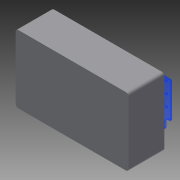
# Autodesk Inventor part: boks
Saved by Autodesk Inventor 2015 (Build 190159000, 159)
## iProperties
Created: 2015-07-23
Part Number: boks
Material: Generic
Document SubType Name: Modeling
Designer: Simen
Density: 1 g/cm^3
Appearance: Default
Author: Simen
Autodesk Inventor part; units mm, degrees
ref_plane "YZ Plane" through (0, 0, 0) normal (1, 0, 0) x (0, 1, 0)
ref_plane "XZ Plane" through (0, 0, 0) normal (0, 1, 0) x (-1, 0, 0)
ref_plane "XY Plane" through (0, 0, 0) normal (0, 0, 1) x (1, 0, 0)
sketch "Sketch1" plane through (0, 0, 0) normal (0, 1, 0) x (-1, 0, 0)
  line L0 (0, 0) -> (200, 0)
  line L1 (200, 0) -> (200, -120)
  line L2 (200, -120) -> (0, -120)
  line L3 (0, -120) -> (0, 0)
  dimension "d0" = 200
  dimension "d1" = 120
  constraints: 8 end point, 2 parallel, 1 horizontal, 1 perpendicular
  measures "d0" distance of L1.end L2.end
  measures "d1" distance of L0.end L1.end
extrude "Extrusion1" add sketch "Sketch1" along normal blind 3
sketch "Sketch2" plane through (0, 3, 0) normal (0, 1, 0) x (1, 0, 0)
  line L0 (-200, 0) -> (0, 0) projected
  line L1 (0, 0) -> (0, 120) projected
  line L2 (0, 120) -> (-200, 120) projected
  line L3 (-200, 120) -> (-200, 0) projected
  line L4 (-181.5, 116.5) -> (-18.5, 116.5)
  line L5 (-3.5, 92.5) -> (-3.5, 27.5)
  line L6 (-18.5, 3.5) -> (-181.5, 3.5)
  line L7 (-196.5, 27.5) -> (-196.5, 92.5)
  line L8 (-196.5, 3.5) -> (-186.5, 3.5)
  line L9 (-186.5, 8.5) -> (-186.5, 17.5)
  line L10 (-191.5, 22.5) -> (-191.5, 22.5)
  line L11 (-196.5, 22.5) -> (-196.5, 3.5)
  line L12 (-196.5, 116.5) -> (-186.5, 116.5)
  line L13 (-186.5, 111.5) -> (-186.5, 102.5)
  line L14 (-191.5, 97.5) -> (-191.5, 97.5)
  line L15 (-196.5, 97.5) -> (-196.5, 116.5)
  line L16 (-3.5, 116.5) -> (-13.5, 116.5)
  line L17 (-13.5, 111.5) -> (-13.5, 102.5)
  line L18 (-8.5, 97.5) -> (-8.5, 97.5)
  line L19 (-3.5, 97.5) -> (-3.5, 116.5)
  line L20 (-3.5, 3.5) -> (-13.5, 3.5)
  line L21 (-13.5, 8.5) -> (-13.5, 17.5)
  line L22 (-8.5, 22.5) -> (-8.5, 22.5)
  line L23 (-3.5, 22.5) -> (-3.5, 3.5)
  arc A0 (-3.5, 92.5) -> (-8.5, 97.5) centre (-8.5, 92.5) ccw
  arc A1 (-13.5, 111.5) -> (-18.5, 116.5) centre (-18.5, 111.5) ccw
  arc A2 (-8.5, 22.5) -> (-3.5, 27.5) centre (-8.5, 27.5) ccw
  arc A3 (-18.5, 3.5) -> (-13.5, 8.5) centre (-18.5, 8.5) ccw
  arc A4 (-186.5, 8.5) -> (-181.5, 3.5) centre (-181.5, 8.5) ccw
  arc A5 (-196.5, 27.5) -> (-191.5, 22.5) centre (-191.5, 27.5) ccw
  arc A6 (-191.5, 97.5) -> (-196.5, 92.5) centre (-191.5, 92.5) ccw
  arc A7 (-181.5, 116.5) -> (-186.5, 111.5) centre (-181.5, 111.5) ccw
  arc A8 (-191.5, 97.5) -> (-186.5, 102.5) centre (-191.5, 102.5) ccw
  arc A9 (-186.5, 17.5) -> (-191.5, 22.5) centre (-191.5, 17.5) ccw
  arc A10 (-8.5, 22.5) -> (-13.5, 17.5) centre (-8.5, 17.5) ccw
  arc A11 (-13.5, 102.5) -> (-8.5, 97.5) centre (-8.5, 102.5) ccw
  line L24 (-196.5, 116.5) -> (-200, 116.5)
  line L25 (-196.5, 3.5) -> (-200, 3.5)
  line L26 (-3.5, 3.5) -> (-3.5, 0)
  line L27 (-3.5, 116.5) -> (-3.5, 120)
  line L28 (-196.5, 3.5) -> (-196.5, 0)
  point P0 (-186.5, 22.5)
  point P1 (-186.5, 97.5)
  point P2 (-13.5, 97.5)
  point P3 (-13.5, 22.5)
  dimension "d4" = 3.5
  dimension "d7" = 10
  dimension "d8" = 19
  dimension "d9" = 10
  dimension "d10" = 19
  dimension "d11" = 10
  dimension "d12" = 19
  dimension "d13" = 10
  dimension "d14" = 19
  dimension "d15" = 5
  dimension "d16" = 5
  dimension "d17" = 5
  dimension "d18" = 5
  dimension "d19" = 5
  dimension "d20" = 5
  dimension "d21" = 5
  dimension "d22" = 5
  dimension "d23" = 5
  dimension "d73" = 3.5
  dimension "d74" = 3.5
  dimension "d75" = 3.5
  dimension "d78" = 3.5
  constraints: 50 end point, 29 point on line, 24 point on circle, 24 tangent, 12 centre point, 8 parallel, 8 perpendicular, 4 horizontal, 3 equal radius, 1 vertical, 1 other
  measures "d4" distance between parallel lines of L2 L4
  measures "d7" distance of L11.start point (-186.5, 22.5)
  measures "d8" distance of L8.end point (-186.5, 22.5)
  measures "d9" distance of point (-186.5, 97.5) L15.start
  measures "d10" distance of L12.end point (-186.5, 97.5)
  measures "d11" distance of L19.start point (-13.5, 97.5)
  measures "d12" distance of point (-13.5, 97.5) L16.end
  measures "d13" distance of point (-13.5, 22.5) L23.start
  measures "d14" distance of L20.end point (-13.5, 22.5)
  measures "d15" radius of A0
  measures "d16" radius of A1
  measures "d17" radius of A2
  measures "d18" radius of A3
  measures "d19" radius of A4
  measures "d20" radius of A5
  measures "d21" radius of A6
  measures "d22" radius of A7
  measures "d23" radius of A8
  measures "d73" distance of L12.start L24.end
  measures "d74" distance of L8.start L25.end
  measures "d75" distance of L20.start L26.end
  measures "d78" distance of L8.start L28.end
extrude "Extrusion2" add sketch "Sketch2" along normal blind 60
sketch "Sketch3" plane through (0, 3, 0) normal (0, 1, 0) x (1, 0, 0)
  line L0 (-200, 120) -> (-200, 105)
  line L1 (-200, 120) -> (-200, 0) projected
  line L2 (0, 120) -> (0, 0) projected
  line L3 (0, 0) -> (0, 15)
  line L4 (-181.5, 3.5) -> (-18.5, 3.5) projected
  circle A0 centre (-180, 105) radius 1.5
  line L5 (-180, 105) -> (-158, 105)
  circle A1 centre (-158, 105) radius 1.5
  circle A2 centre (-187.5, 60) radius 1.5
  line L6 (-187.5, 60) -> (-187.5, 80)
  line L7 (-187.5, 60) -> (-187.5, 40)
  circle A3 centre (-187.5, 40) radius 1.5
  circle A4 centre (-187.5, 80) radius 1.5
  line L8 (-200, 0) -> (-200, 120) projected
  line L9 (-187.5, 60) -> (-12.5, 60)
  circle A5 centre (-12.5, 60) radius 1.5
  line L10 (0, 120) -> (-200, 120) projected
  line L11 (-100, 120) -> (-100, 0)
  line L12 (0, 0) -> (-200, 0) projected
  circle A6 centre (-20, 105) radius 1.5
  line L13 (-180, 105) -> (-181.5, 105)
  line L14 (-184, 106) -> (-200, 106)
  line L15 (-180, 105) -> (-159.5, 105)
  line L16 (-180, 15) -> (-20, 15)
  circle A7 centre (-180, 15) radius 1.5
  line L17 (-84.857, 105) -> (-84.857, 15)
  line L18 (-158, 105) -> (-20, 105)
  circle A8 centre (-20, 15) radius 1.5
  line L19 (-12.5, 60) -> (-12.5, 40)
  line L20 (-12.5, 60) -> (-12.5, 80)
  circle A9 centre (-12.5, 80) radius 1.5
  circle A10 centre (-12.5, 40) radius 1.5
  line L21 (-180, 105) -> (-20, 105)
  line L22 (-13.5, 111.5) -> (-13.5, 102.5) projected
  point P0 (-100, 60)
  point P1 (-100, 15)
  point P2 (-84.857, 60)
  point P3 (-100, 105)
  dimension "d35" = 3
  dimension "d37" = 3
  dimension "d24" = 15
  dimension "d36" = 22
  dimension "d41" = 3
  dimension "d44" = 20
  dimension "d45" = 20
  dimension "d54" = 175
  dimension "d55" = 3
  dimension "d57" = 3
  dimension "d59" = 160
  dimension "d60" = 3
  dimension "d62" = 90
  dimension "d63" = 3
  dimension "d64" = 20
  dimension "d65" = 20
  dimension "d66" = 3
  dimension "d67" = 3
  dimension "d68" = 3
  dimension "d69" = 3
  dimension "d72" = 138
  constraints: 32 end point, 9 centre point, 8 coincident, 8 point on line, 7 midpoint, 6 perpendicular, 4 vertical, 3 horizontal, 2 horizontal alignment, 4 other
  measures "d24" distance of L0.start L0.end
  measures "d36" distance of L5.start L5.end
  measures "d41" diameter of A2
  measures "d44" distance of L6.start L6.end
  measures "d45" distance of L6.start L7.end
  measures "d54" distance of L6.start L9.end
  measures "d55" diameter of A5
  measures "d57" diameter of A6
  measures "d59" distance of L16.start L16.end
  measures "d60" diameter of A7
  measures "d62" distance of L17.start L17.end
  measures "d63" diameter of A8
  measures "d64" distance of L19.start L19.end
  measures "d65" distance of L19.start L20.end
  measures "d66" diameter of A9
  measures "d67" diameter of A10
  measures "d68" diameter of A4
  measures "d69" diameter of A3
  measures "d72" distance of L18.start L18.end
fillet "Fillet2" radius 5 4 edges at (0, 31.5, 0) (0, 31.5, -120) (-200, 31.5, -120) (-200, 31.5, 0)
extrude "Extrusion4" add sketch "Sketch3" along normal blind 5.6 contours A7 | A3 | A4 | A2 L7 L9 | L9 L6 A2 | A0 L13 L5 | L5 L13 A0 | A1 L5 L18 | L18 L5 A1 | A6 | A9 | A10 | A5 L20 L9 | L9 L19 A5 | A8 | L6 L7 A2 | L20 A5 L19
body "Solid1"
